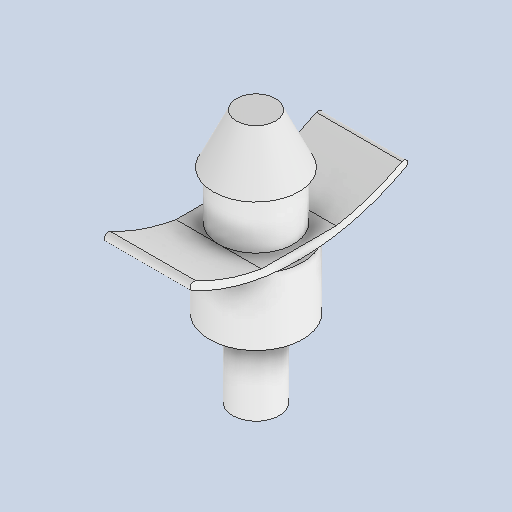
# Autodesk Inventor part: WBN-305
Saved by Autodesk Inventor 2024.2 (Build 282272000, 272)
## iProperties
Created: 2024-01-25
Part Number: WBN-305
Material: Acetal Resin, White
Document SubType Name: Modeling
Designer: Masato Kubotera
Density: 1.425 g/cm^3
Appearance: Smooth - White
Vendor: HIROSUGI
Catalog Web Link: https://www.hirosugi-net.co.jp/shop/g/g107030/
Author: Masato Kubotera
Autodesk Inventor part; units mm, degrees
ref_plane "YZ Plane" through (0, 0, 0) normal (1, 0, 0) x (0, 1, 0)
ref_plane "XZ Plane" through (0, 0, 0) normal (0, 1, 0) x (-1, 0, 0)
ref_plane "XY Plane" through (0, 0, 0) normal (0, 0, 1) x (1, 0, 0)
sketch "Sketch1" plane through (0, 0, 0) normal (0, 1, 0) x (-1, 0, 0)
  line L0 (0, 0) -> (0, 16.2928)
  line L1 (0, 16.2928) -> (-1.2578, 16.2928)
  line L2 (-1.2578, 16.2928) -> (-2.75, 13.0928)
  line L3 (-2.75, 13.0928) -> (-2.4, 13.0928)
  line L4 (-2.4, 13.0928) -> (-2.4, 9.2928)
  line L5 (-2.4, 9.2928) -> (-3, 9.2928)
  line L6 (-3, 9.2928) -> (-3, 5)
  line L7 (-3, 5) -> (-1.5, 5)
  line L8 (-1.5, 5) -> (-1.5, 0)
  line L9 (-1.5, 0) -> (0, 0)
  arc A0 (-6.8684, 11.0226) -> (0, 9.2928) centre (0, 23.7935) ccw
  arc A1 (-6.6316, 11.4629) -> (-2.4, 10) centre (0, 23.7935) ccw
  arc A2 (-6.6316, 11.4629) -> (-6.8684, 11.0226) centre (-6.75, 11.2428) ccw
  line L10 (-2.4, 10) -> (0, 10)
  point P0 (0, 10)
  dimension "d0" = 3
  dimension "d1" = 5
  dimension "d3" = 6
  dimension "d4" = 3.2
  dimension "d5" = 5.5
  dimension "d9" = 7
  dimension "d10" = 25
  dimension "d11" = 4.8
  dimension "d15" = 5
  dimension "d17" = 14
  dimension "d18" = 0.5
  dimension "d19" = 1.6
  constraints: 22 end point, 6 point on circle, 5 point on line, 4 horizontal, 4 vertical, 3 centre point, 3 tangent, 1 coincident, 1 perpendicular
  measures "d0" diameter of L8 L0
  measures "d1" distance of L7.end L8.end
  measures "d3" diameter of L6 L0
  measures "d4" distance between parallel lines of L3 L1
  measures "d5" diameter of L2.end L0
  measures "d9" distance between parallel lines of L5 L1
  measures "d10" angle of L2 L0
  measures "d11" diameter of L4 L0
  measures "d15" distance between parallel lines of L7 L10
  measures "d18" radial gap between concentric circles of A0 A1
  measures "d19" distance edge to line of A2 L3
revolve "Revolution1" add sketch "Sketch1" angle 360 about axis through (0, 0, 0) along (0, 0, 1) contours L9 L8 L7 L6 L5 L4 A0 L0 | A0 L4 L10 L0 | L10 L4 L3 L2 L1 L0
extrude "Extrusion1" add sketch "Sketch1" along normal mid plane 5.5 contours A0 L4 L10 L0 | A0 A2 A1 L4
mirror "Mirror1" about plane through (0, 0, 9.2928) normal (-1, 0, 0) of "Extrusion1"
body "Solid1"
